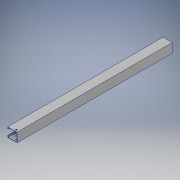
# Autodesk Inventor part: TelescopeMiddleNoSlot
Saved by Autodesk Inventor 2018.3 (Build 223284000, 284)
## iProperties
Created: 2020-01-18
Part Number: TelescopeMiddleNoSlot
Material: Aluminum 6061
Document SubType Name: Modeling
Designer: Cooper
Density: 2.7 g/cm^3
Appearance: Aluminum - Flat
Mass: 274.138 g
Surface Area: 1283.56 cm^2
Volume: 101.533 cm^3
Author: Cooper
Autodesk Inventor part; units mm, degrees
ref_plane "XZ Plane" through (0, 0, 0) normal (0, 1, 0) x (-1, 0, 0)
ref_plane "XY Plane" through (0, 0, 0) normal (0, 0, 1) x (1, 0, 0)
sketch "Sketch1" plane through (0, 0, 0) normal (0, 0, 1) x (1, 0, 0)
  line L0 (0, 0) -> (31.75, 0)
  line L1 (31.75, 0) -> (31.75, 31.75)
  line L2 (31.75, 31.75) -> (0, 31.75)
  line L3 (0, 31.75) -> (0, 0)
  line L4 (1.5875, 30.1625) -> (30.1625, 30.1625)
  line L5 (30.1625, 30.1625) -> (30.1625, 1.5875)
  line L6 (30.1625, 1.5875) -> (1.5875, 1.5875)
  line L7 (1.5875, 1.5875) -> (1.5875, 30.1625)
  dimension "d0" = 31.75
  dimension "d1" = 31.75
  dimension "d2" = 1.5875
  constraints: 16 end point, 4 parallel, 2 perpendicular, 1 horizontal, 3 other
  measures "d0" distance of L2.end L0.start
  measures "d1" distance of L0.start L0.end
  measures "d2" distance between parallel lines of L2 L4
extrude "Extrusion1" add sketch "Sketch1" along normal blind 533.4
sketch "Sketch5" plane through (31.75, 0, 0) normal (1, 0, 0) x (0, 0, -1)
  line L0 (0, 15.875) -> (-12.7, 15.875) construction
  line L1 (0, 6.35) -> (-12.7, 6.35)
  line L2 (-12.7, 25.4) -> (0, 25.4)
  arc A0 (0, 6.35) -> (0, 25.4) centre (0, 15.875) ccw
  arc A1 (-12.7, 25.4) -> (-12.7, 6.35) centre (-12.7, 15.875) ccw
  line L3 (0, 0) -> (0, 31.75) projected
  line L4 (0, 31.75) -> (-533.4, 31.75) projected
  point P0 (-6.35, 15.875)
  dimension "d26" = 0
  dimension "d27" = 19.05
  dimension "d28" = 15.875
  dimension "d29" = 12.7
  constraints: 8 end point, 4 point on circle, 4 tangent, 2 centre point, 1 horizontal, 1 midpoint, 1 parallel, 1 other
  measures "d27" distance between parallel lines of L1 L2
  measures "d28" distance from line of L4 point (-6.35, 15.875)
  measures "d29" distance of L1.start L1.end
extrude "Extrusion4" cut sketch "Sketch5" against normal blind 25.4
ref_plane "Work Plane3" through (15.875, 0, 0) normal (1, 0, 0) x (0, 1, 0)
mirror "Mirror1" about plane through (15.875, 0, 0) normal (1, 0, 0) of "Extrusion4"
sketch "Sketch6" plane through (31.75, 0, 533.4) normal (1, 0, 0) x (0, 0, -1)
  line L0 (533.4, 25.4) -> (520.7, 25.4) projected
  line L1 (533.4, 25.4) -> (520.7, 25.4)
  arc A0 (520.7, 25.4) -> (520.7, 6.35) centre (520.7, 15.875) ccw projected
  arc A1 (520.7, 25.4) -> (520.7, 6.35) centre (520.7, 15.875) ccw
  line L2 (533.4, 6.35) -> (520.7, 6.35) projected
  line L3 (520.7, 6.35) -> (533.4, 6.35)
  line L4 (533.4, 25.4) -> (533.4, 31.75) projected
  line L5 (533.4, 25.4) -> (533.4, 6.35)
  point P0 (533.4, 0)
  constraints: 6 end point, 2 collinear, 2 point on circle, 1 centre point, 1 horizontal, 1 tangent
extrude "Extrusion5" add sketch "Sketch6" against normal blind 1.5875
sketch "Sketch8" plane through (0, 31.75, 0) normal (0, 1, 0) x (1, 0, 0)
  line L0 (31.75, 0) -> (31.75, -533.4) projected
  line L1 (31.75, -533.4) -> (0, -533.4) projected
  point P0 (0, 0)
  point P1 (23.0188, -527.05)
  dimension "d44" = 8.7312
  dimension "d45" = 6.35
  measures "d44" distance from line of L0 point (23.019, -527.05)
  measures "d45" distance from line of L1 point (23.019, -527.05)
hole "Hole3" at (23.0187, 31.75, 527.05) direction (0, -1, 0) diameter 5.1562 depth 76.2 tip angle 118
sketch "Sketch9" plane through (0, 0, 533.4) normal (-1, 0, 0) x (0, 0, 1)
  line L0 (0, 1.5875) -> (0, 30.1625) projected
  line L1 (0, 25.4) -> (-25.4, 25.4)
  line L2 (-25.4, 25.4) -> (-25.4, 6.35)
  line L3 (-25.4, 6.35) -> (0, 6.35)
  line L4 (0, 6.35) -> (0, 25.4)
  line L5 (-533.4, 0) -> (0, 0) projected
  line L6 (-533.4, 31.75) -> (0, 31.75) projected
  dimension "d53" = 25.4
  dimension "d54" = 6.35
  dimension "d55" = 6.35
  constraints: 8 end point, 2 parallel, 1 horizontal, 1 perpendicular, 1 point on line
  measures "d53" distance between parallel lines of L2 L0
  measures "d54" distance between parallel lines of L5 L3
  measures "d55" distance between parallel lines of L6 L1
extrude "Extrusion6" cut sketch "Sketch9" against normal blind 5.842
equation "\"d55\" = d54"
body "Solid1"
